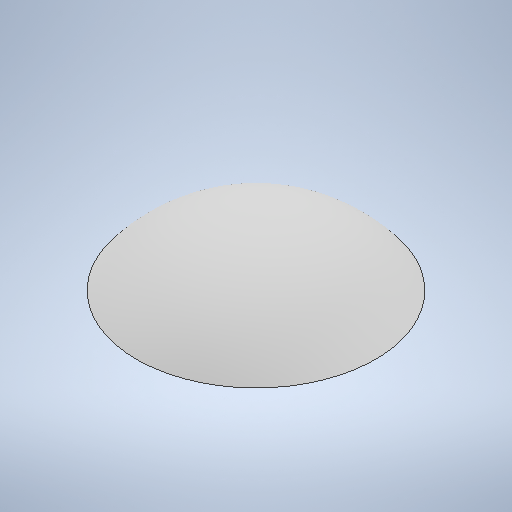
# Autodesk Inventor part: Foot
Saved by Autodesk Inventor 2026.2 (Build 302298000, 298)
## iProperties
Created: 2026-05-09
Part Number: Foot
Material: Generic
Document SubType Name: Modeling
Designer: gaoet
Density: 1 g/cm^3
Appearance: Default
Author: gaoet
Autodesk Inventor part; units mm, degrees
ref_plane "YZ Plane" through (0, 0, 0) normal (1, 0, 0) x (0, 1, 0)
ref_plane "XZ Plane" through (0, 0, 0) normal (0, 1, 0) x (-1, 0, 0)
ref_plane "XY Plane" through (0, 0, 0) normal (0, 0, 1) x (1, 0, 0)
sketch "Sketch1" plane through (0, 0, 0) normal (0, 0, 1) x (1, 0, 0)
  circle A0 centre (0, 0) radius 5
  line L0 (-4, 3) -> (4, 3)
  line L1 (0, 3) -> (0, 5)
  dimension "d0" = 8
  dimension "d3" = 2
  constraints: 4 end point, 3 point on circle, 1 centre point, 1 coincident, 1 horizontal, 1 midpoint, 1 vertical, 1 vertical alignment
  measures "d0" distance of L0.start L0.end
  measures "d3" distance of L1.end L1.start
revolve "Revolution1" add sketch "Sketch1" angle 360 about axis through (0, 3, 0) along (0, 1, 0) picked at (-2.4012, 3.2796) contours A0 L1 L0
body "Solid1"
